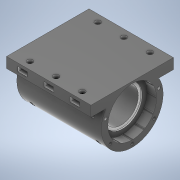
# Autodesk Inventor part: двухопорный корпус
Saved by Autodesk Inventor 2022 (Build 260153000, 153)
## iProperties
Created: 2022-12-27
Part Number: двухопорный корпус
Material: Типовые
Document SubType Name: Modeling
Designer: Pavel
Density: 1 g/cm^3
Appearance: По умолчанию
Author: Pavel
Autodesk Inventor part; units mm, degrees
note: some values were not read from the file. Chosen so that the rebuilt part matches the saved one: pattern direction of "Круговой массив1".
sketch "Эскиз2" plane through (0, 0, 0) normal (1, 0, 0) x (0, 1, 0)
  circle A0 centre (0, 0) radius 13
  circle A1 centre (0, 0) radius 18.65
  dimension "d0" = 26
  dimension "d1" = 37.3
  constraints: 2 centre point, 2 coincident
  measures "d0" diameter of A0
  measures "d1" diameter of A1
extrude "Выдавливание1" add sketch "Эскиз2" along normal blind 50
sketch "Эскиз3" plane through (50, 0, 0) normal (1, 0, 0) x (0, 0, -1)
  circle A0 centre (0, 0) radius 18.65 projected
  circle A1 centre (0, 0) radius 18.65
  arc A2 (-12.4624, 20.1) -> (12.4624, 20.1) centre (0, 0) ccw
  line L0 (12.4624, 20.1) -> (-12.4624, 20.1)
  dimension "d4" = 0
  dimension "d5" = 5
  dimension "d50" = 20.1
  constraints: 2 centre point, 2 coincident, 2 end point, 2 point on circle, 1 horizontal
  measures "d4" radial gap between concentric circles of A0 A1
  measures "d5" radial gap between concentric circles of A0 A2
  measures "d50" distance from line of L0 point (0, 0)
extrude "Выдавливание2" add sketch "Эскиз3" along normal blind 7.3 and the other way blind 57.3
sketch "Эскиз4" plane through (57.3, 0, 0) normal (1, 0, 0) x (0, 0, -1)
  arc A0 (-12.4624, 20.1) -> (12.4624, 20.1) centre (0, 0) ccw projected
  circle A1 centre (0, 0) radius 18.65 projected
  line L0 (0, -23.65) -> (0, -18.65) construction
  circle A2 centre (0, -21.15) radius 1.1
  dimension "d11" = 2.2
  constraints: 2 end point, 2 midpoint, 1 centre point, 1 point on circle, 1 vertical, 1 vertical alignment, 1 other
  measures "d11" diameter of A2
extrude "Выдавливание3" cut sketch "Эскиз4" against normal blind 13 contours A2
ref_plane "РабПлоскость2" through (50.3, 0, 0) normal (1, 0, 0) x (0, 0, -1)
sketch "Эскиз5" plane through (50.3, 0, 0) normal (1, 0, 0) x (0, 0, -1)
  line L0 (-2.1, -22.3624) -> (-2.1, -19.9376)
  line L1 (-2.1, -19.9376) -> (0, -18.7251)
  line L2 (0, -18.7251) -> (2.1, -19.9376)
  line L3 (2.1, -19.9376) -> (2.1, -22.3624)
  circle A0 centre (0, -21.15) radius 1.1 projected
  line L4 (2.1, -22.3624) -> (2.1, -23.5566)
  arc A1 (-12.4624, 20.1) -> (12.4624, 20.1) centre (0, 0) ccw projected
  line L5 (-2.1, -22.3624) -> (-2.1, -23.5566)
  dimension "d16" = 4.2
  constraints: 12 end point, 2 coincident, 2 point on circle, 2 vertical, 1 parallel, 8 other
  measures "d16" distance between parallel lines of L0 L3
extrude "Выдавливание4" cut sketch "Эскиз5" along normal mid plane 1.7
pattern_circular "Круговой массив1" count 5 over 210 about axis through (50, 0, 0) along (1, 0, 0) of "Выдавливание3", "Выдавливание4" both ways yes
ref_plane "РабПлоскость3" through (25, 0, 0) normal (1, 0, 0) x (0, 0, -1)
mirror "Зеркальное отражение1" about plane through (25, 0, 0) normal (1, 0, 0) of "Выдавливание3", "Выдавливание4", "Круговой массив1"
sketch "Эскиз6" plane through (-7.3, 20.1, 12.4624) normal (0, 1, 0) x (1, 0, 0)
  line L0 (0, 0) -> (64.6, 0) projected
  line L1 (64.6, 24.9249) -> (64.6, 0) construction
  line L2 (64.6, 24.9249) -> (0, 24.9249) construction
  line L3 (0, 0) -> (0, 24.9249) construction
  line L4 (64.6, 24.9249) -> (0, 24.9249) projected
  line L5 (64.6, 24.9249) -> (64.6, 0) projected
  line L6 (0, 24.9249) -> (64.6, 0) construction
  line L7 (0, -19.0876) -> (64.6, -19.0876)
  line L8 (64.6, -19.0876) -> (64.6, 44.0124)
  line L9 (64.6, 44.0124) -> (0, 44.0124)
  line L10 (0, 44.0124) -> (0, -19.0876)
  line L11 (0, -19.0876) -> (64.6, 44.0124) construction
  line L12 (64.6, -19.0876) -> (0, 44.0124) construction
  point P0 (32.3, 12.4624)
  point P1 (0, 24.9249)
  point P2 (64.6, 24.9249)
  dimension "d22" = 63.1
  constraints: 14 end point, 3 midpoint, 2 parallel, 1 collinear, 1 horizontal, 1 perpendicular
  measures "d22" distance between parallel lines of L7 L9
extrude "Выдавливание5" add sketch "Эскиз6" against normal blind 8 contours L0 L8 L7 L10 | L10 L9 L8 L4
sketch "Эскиз7" plane through (-7.3, 12.1, 12.4624) normal (0, -1, 0) x (1, 0, 0)
  line L0 (64.6, 7.8578) -> (0, 7.8578) construction
  line L1 (0, 19.0876) -> (0, 7.8578) construction
  line L2 (0, 13.4727) -> (64.6, 13.4727) construction
  line L3 (64.6, 7.8578) -> (64.6, 19.0876) construction
  line L4 (7.3, -12.4624) -> (57.3, -12.4624) construction
  line L5 (57.3, -24.9249) -> (57.3, 0) construction
  circle A0 centre (12.3, 13.4727) radius 2.1
  circle A1 centre (32.3, 13.4727) radius 2.1
  circle A2 centre (52.3, 13.4727) radius 2.1
  circle A3 centre (12.3, -38.3976) radius 2.1
  circle A4 centre (32.3, -38.3976) radius 2.1
  circle A5 centre (52.3, -38.3976) radius 2.1
  dimension "d25" = 20
  dimension "d26" = 20
  dimension "d27" = 4.2
  constraints: 6 centre point, 4 end point, 4 midpoint, 3 symmetric about line, 2 equal radius, 2 point on line, 3 other
  measures "d25" distance of A1.centre A0.centre
  measures "d26" distance of A2.centre A1.centre
  measures "d27" diameter of A0
extrude "Выдавливание6" cut sketch "Эскиз7" against normal up to surface (8 mm away)
ref_plane "РабПлоскость4" through (-10.3, -23.65, -23.65) normal (-1, 0, 0) x (0, 0, 1)
sketch "Эскиз9" plane through (-7.3, 0, 0) normal (-1, 0, 0) x (0, 0, 1)
  circle A0 centre (0, -18.65) radius 0.25
  line L0 (0, 0) -> (0, -18.65) construction
  dimension "d40" = 0.5
  dimension "d43" = 18.65
  constraints: 2 end point, 1 centre point, 1 vertical
  measures "d40" diameter of A0
  measures "d43" distance of L0.start L0.end
extrude "Выдавливание9" add sketch "Эскиз9" against normal up to surface (7.3 mm away)
fillet "Сопряжение1" radius 0.7 2 edges at (-3.65, -18.6483, -0.25) (-3.65, -18.6483, 0.25)
pattern_circular "Круговой массив2" count 12 over 360 about axis through (0, 0, 0) along (1, 0, 0) of "Выдавливание9", "Сопряжение1"
mirror "Зеркальное отражение2" about plane through (25, 0, 0) normal (1, 0, 0) of "Выдавливание9", "Сопряжение1", "Круговой массив2"
sketch "Эскиз10" plane through (-7.3, 0, 0) normal (-1, 0, 0) x (0, 0, 1)
  arc A0 (-16.4687, 8.7524) -> (-18.6385, 0.6546) centre (0, 0) ccw projected
  circle A1 centre (0, 0) radius 18.65
  line L0 (-12.4624, 12.1) -> (-14.192, 12.1) projected
  line L1 (-12.4624, 12.1) -> (-14.192, 12.1)
  line L2 (-12.4624, 13.8748) -> (-12.4624, 12.1) projected
  line L3 (-14.192, 12.1) -> (-12.4624, 12.1)
  line L4 (-12.4624, 12.1) -> (-12.4624, 13.8748)
  line L5 (14.192, 12.1) -> (12.4624, 12.1) projected
  arc A2 (12.4624, 13.8748) -> (9.8861, 15.8141) centre (0, 0) ccw projected
  line L6 (12.4624, 12.1) -> (12.4624, 13.8748)
  line L7 (12.4624, 13.8748) -> (12.4624, 12.1)
  line L8 (14.192, 12.1) -> (12.4624, 12.1)
  constraints: 12 end point, 4 collinear, 1 coincident, 1 perpendicular, 1 vertical, 4 other
extrude "Выдавливание10" cut sketch "Эскиз10" against normal up to surface (7.3 mm away) contours A1 L2 L0 | L5 L6 A1
mirror "Зеркальное отражение3" about plane through (25, 0, 0) normal (1, 0, 0) of "Выдавливание10"
ref_plane "РабПлоскость5" through (-7.3, 16.1, 12.4624) normal (0, -1, 0) x (1, 0, 0)
sketch "Эскиз11" plane through (-7.3, 16.1, 12.4624) normal (0, -1, 0) x (1, 0, 0)
  circle A0 centre (12.3, 13.4727) radius 2.1 projected
  circle A1 centre (12.3, 13.4727) radius 2.1 projected
  line L0 (12.3, 9.3735) -> (8.75, 11.4231)
  line L1 (8.75, 11.4231) -> (8.75, 15.5223)
  line L2 (8.75, 15.5223) -> (12.3, 17.5719)
  line L3 (12.3, 17.5719) -> (15.85, 15.5223)
  line L4 (15.85, 15.5223) -> (15.85, 11.4231)
  line L5 (15.85, 11.4231) -> (12.3, 9.3735)
  line L6 (0, -44.0124) -> (0, 19.0876) construction
  line L7 (0, -44.0124) -> (0, 19.0876)
  line L8 (0, 19.0876) -> (64.6, 19.0876) construction
  line L9 (64.6, -12.4624) -> (0, -12.4624) construction
  line L10 (32.3, 9.3735) -> (28.75, 11.4231)
  line L11 (28.75, 11.4231) -> (28.75, 15.5223)
  line L12 (28.75, 15.5223) -> (32.3, 17.5719)
  line L13 (32.3, 17.5719) -> (35.85, 15.5223)
  line L14 (35.85, 15.5223) -> (35.85, 11.4231)
  line L15 (35.85, 11.4231) -> (32.3, 9.3735)
  line L16 (52.3, 9.3735) -> (48.75, 11.4231)
  line L17 (48.75, 11.4231) -> (48.75, 15.5223)
  line L18 (48.75, 15.5223) -> (52.3, 17.5719)
  line L19 (52.3, 17.5719) -> (55.85, 15.5223)
  line L20 (55.85, 15.5223) -> (55.85, 11.4231)
  line L21 (55.85, 11.4231) -> (52.3, 9.3735)
  circle A2 centre (12.3, -38.3976) radius 2.1
  circle A3 centre (12.3, -38.3976) radius 2.1
  line L22 (12.3, -34.2984) -> (8.75, -36.348)
  line L23 (8.75, -36.348) -> (8.75, -40.4472)
  line L24 (8.75, -40.4472) -> (12.3, -42.4968)
  line L25 (12.3, -42.4968) -> (15.85, -40.4472)
  line L26 (15.85, -40.4472) -> (15.85, -36.348)
  line L27 (15.85, -36.348) -> (12.3, -34.2984)
  line L28 (32.3, -34.2984) -> (28.75, -36.348)
  line L29 (28.75, -36.348) -> (28.75, -40.4472)
  line L30 (28.75, -40.4472) -> (32.3, -42.4968)
  line L31 (32.3, -42.4968) -> (35.85, -40.4472)
  line L32 (35.85, -40.4472) -> (35.85, -36.348)
  line L33 (35.85, -36.348) -> (32.3, -34.2984)
  line L34 (52.3, -34.2984) -> (48.75, -36.348)
  line L35 (48.75, -36.348) -> (48.75, -40.4472)
  line L36 (48.75, -40.4472) -> (52.3, -42.4968)
  line L37 (52.3, -42.4968) -> (55.85, -40.4472)
  line L38 (55.85, -40.4472) -> (55.85, -36.348)
  line L39 (55.85, -36.348) -> (52.3, -34.2984)
  line L40 (0, -44.0124) -> (64.6, -44.0124) projected
  line L41 (64.6, -44.0124) -> (0, -44.0124)
  line L42 (64.6, -44.0124) -> (64.6, 19.0876)
  line L43 (59.9835, -44.0124) -> (59.9835, -12.4624) construction
  line L44 (60.9342, -12.4624) -> (60.9342, 19.0876) construction
  line L45 (64.6, 19.0876) -> (0, 19.0876) projected
  line L46 (55.85, 15.5223) -> (55.85, 19.0876)
  line L47 (48.75, 15.5223) -> (48.75, 19.0876)
  line L48 (35.85, 15.5223) -> (35.85, 19.0876)
  line L49 (28.75, 15.5223) -> (28.75, 19.0876)
  line L50 (15.85, 15.5223) -> (15.85, 19.0876)
  line L51 (8.75, 15.5223) -> (8.75, 19.0876)
  line L52 (55.85, -40.4472) -> (55.85, -44.0124)
  line L53 (48.75, -40.4472) -> (48.75, -44.0124)
  line L54 (35.85, -40.4472) -> (35.85, -44.0124)
  line L55 (28.75, -40.4472) -> (28.75, -44.0124)
  line L56 (15.85, -40.4472) -> (15.85, -44.0124)
  line L57 (8.75, -40.4472) -> (8.75, -44.0124)
  point P0 (7.3, -12.4624)
  point P1 (32.3, 13.4727)
  point P2 (52.3, 13.4727)
  point P3 (32.3, -38.3976)
  point P4 (52.3, -38.3976)
  point P5 (35.85, 19.0876)
  point P6 (28.75, 19.0876)
  point P7 (15.85, 19.0876)
  point P8 (8.75, 19.0876)
  point P9 (8.75, 15.5223)
  dimension "d53" = 7.1
  dimension "d63" = 20
  dimension "d70" = 20
  constraints: 110 end point, 33 symmetric about line, 7 perpendicular, 6 point on line, 2 centre point, 2 coincident, 2 horizontal, 2 vertical, 1 collinear, 1 midpoint, 1 parallel, 53 other
  measures "d53" distance between parallel lines of L1 L4
  measures "d63" distance of point (12.3, 13.473) point (32.3, 13.473)
  measures "d70" distance of L19.end L48.start
extrude "Выдавливание11" cut sketch "Эскиз11" along normal mid plane 3.5 contours A0 | L0 L1 L2 L3 L4 L5 | L51 L45 L50 L3 L2 | L45 L48 L13 L12 L49 | L12 L13 L14 L15 L10 L11 | L57 L24 L25 L56 L40 | L45 L46 L19 L18 L47 | L23 L22 L27 L26 L25 L24 | L18 L19 L20 L21 L16 L17 | L55 L30 L31 L54 L40 | L29 L28 L33 L32 L31 L30 | L53 L36 L37 L52 L40 | L35 L34 L39 L38 L37 L36 | A2
sketch "Эскиз12" plane through (50, 0, 0) normal (1, 0, 0) x (0, 0, -1)
  circle A0 centre (0, 0) radius 13 projected
  circle A1 centre (0, 0) radius 15
  dimension "d77" = 2
  constraints: 1 centre point, 1 coincident
  measures "d77" radial gap between concentric circles of A0 A1
extrude "Выдавливание12" cut sketch "Эскиз12" against normal blind 1
mirror "Зеркальное отражение4" about plane through (25, 0, 0) normal (1, 0, 0) of "Выдавливание12"
sketch "Эскиз8" plane through (-7.3, 12.1, 12.4624) normal (0, -1, 0) x (1, 0, 0)
  circle A0 centre (12.3, 13.4727) radius 2.1 projected
  line L0 (8.1719, 13.4727) -> (10.236, 17.0477)
  line L1 (10.236, 17.0477) -> (14.364, 17.0477)
  line L2 (14.364, 17.0477) -> (16.4281, 13.4727)
  line L3 (16.4281, 13.4727) -> (14.364, 9.8977)
  line L4 (14.364, 9.8977) -> (10.236, 9.8977)
  line L5 (10.236, 9.8977) -> (8.1719, 13.4727)
  line L6 (28.1719, 13.4727) -> (30.236, 17.0477)
  line L7 (30.236, 17.0477) -> (34.364, 17.0477)
  line L8 (34.364, 17.0477) -> (36.4281, 13.4727)
  line L9 (36.4281, 13.4727) -> (34.364, 9.8977)
  line L10 (34.364, 9.8977) -> (30.236, 9.8977)
  line L11 (30.236, 9.8977) -> (28.1719, 13.4727)
  line L12 (48.1719, 13.4727) -> (50.236, 17.0477)
  line L13 (50.236, 17.0477) -> (54.364, 17.0477)
  line L14 (54.364, 17.0477) -> (56.4281, 13.4727)
  line L15 (56.4281, 13.4727) -> (54.364, 9.8977)
  line L16 (54.364, 9.8977) -> (50.236, 9.8977)
  line L17 (50.236, 9.8977) -> (48.1719, 13.4727)
  line L18 (7.3, -12.4624) -> (57.3, -12.4624) construction
  line L19 (57.3, -24.9249) -> (57.3, 0) construction
  circle A1 centre (12.3, -38.3976) radius 2.1
  line L20 (8.1719, -38.3976) -> (10.236, -41.9726)
  line L21 (10.236, -41.9726) -> (14.364, -41.9726)
  line L22 (14.364, -41.9726) -> (16.4281, -38.3976)
  line L23 (16.4281, -38.3976) -> (14.364, -34.8226)
  line L24 (14.364, -34.8226) -> (10.236, -34.8226)
  line L25 (10.236, -34.8226) -> (8.1719, -38.3976)
  line L26 (28.1719, -38.3976) -> (30.236, -41.9726)
  line L27 (30.236, -41.9726) -> (34.364, -41.9726)
  line L28 (34.364, -41.9726) -> (36.4281, -38.3976)
  line L29 (36.4281, -38.3976) -> (34.364, -34.8226)
  line L30 (34.364, -34.8226) -> (30.236, -34.8226)
  line L31 (30.236, -34.8226) -> (28.1719, -38.3976)
  line L32 (48.1719, -38.3976) -> (50.236, -41.9726)
  line L33 (50.236, -41.9726) -> (54.364, -41.9726)
  line L34 (54.364, -41.9726) -> (56.4281, -38.3976)
  line L35 (56.4281, -38.3976) -> (54.364, -34.8226)
  line L36 (54.364, -34.8226) -> (50.236, -34.8226)
  line L37 (50.236, -34.8226) -> (48.1719, -38.3976)
  point P0 (32.3, 13.4727)
  point P1 (32.3, 13.4727)
  point P2 (52.3, 13.4727)
  point P3 (52.3, 13.4727)
  point P4 (32.3, -38.3976)
  point P5 (32.3, -38.3976)
  point P6 (52.3, -38.3976)
  point P7 (52.3, -38.3976)
  dimension "d30" = 7.15
  dimension "d33" = 20
  constraints: 74 end point, 24 symmetric about line, 6 coincident, 2 horizontal, 1 centre point, 1 collinear, 1 midpoint, 41 other
  measures "d30" distance between parallel lines of L1 L4
  measures "d33" distance of point (12.3, 13.473) point (32.3, 13.473)
